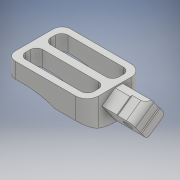
# Autodesk Inventor part: FootpegLeft
Saved by Autodesk Inventor 2018 (Build 220112000, 112)
## iProperties
Created: 2018-01-01
Part Number: FootpegLeft
Material: Generic
Document SubType Name: Modeling
Designer: eroldan
Density: 1 g/cm^3
Appearance: Default
Author: eroldan
Autodesk Inventor part; units mm, degrees
ref_plane "YZ Plane" through (0, 0, 0) normal (1, 0, 0) x (0, 1, 0)
ref_plane "XZ Plane" through (0, 0, 0) normal (0, 1, 0) x (-1, 0, 0)
ref_plane "XY Plane" through (0, 0, 0) normal (0, 0, 1) x (1, 0, 0)
sketch "Sketch1" plane through (0, 0, 0) normal (0, 0, 1) x (1, 0, 0)
  line L0 (-32.5, -28.6) -> (29.5, -28.6)
  line L1 (41.5, -16.6) -> (41.5, 16.6)
  line L2 (29.5, 28.6) -> (-32.5, 28.6)
  line L3 (-41.5, 19.6) -> (-41.5, -19.6)
  line L4 (-41.5, -28.6) -> (41.5, 28.6) construction
  line L5 (41.5, -28.6) -> (-41.5, 28.6) construction
  arc A0 (-32.5, 28.6) -> (-41.5, 19.6) centre (-32.5, 19.6) ccw
  arc A1 (-41.5, -19.6) -> (-32.5, -28.6) centre (-32.5, -19.6) ccw
  arc A2 (41.5, 16.6) -> (29.5, 28.6) centre (29.5, 16.6) ccw
  arc A3 (29.5, -28.6) -> (41.5, -16.6) centre (29.5, -16.6) ccw
  line L6 (-28.5, 21.72) -> (28.5, 21.72)
  line L7 (35, 15.22) -> (35, 10.62)
  line L8 (28.5, 4.12) -> (-28.5, 4.12)
  line L9 (-35, 10.62) -> (-35, 15.22)
  line L10 (-35, 21.72) -> (35, 4.12) construction
  line L11 (35, 21.72) -> (-35, 4.12) construction
  arc A4 (-28.5, 21.72) -> (-35, 15.22) centre (-28.5, 15.22) ccw
  arc A5 (35, 15.22) -> (28.5, 21.72) centre (28.5, 15.22) ccw
  arc A6 (28.5, 4.12) -> (35, 10.62) centre (28.5, 10.62) ccw
  arc A7 (-35, 10.62) -> (-28.5, 4.12) centre (-28.5, 10.62) ccw
  line L12 (-57.2181, 0) -> (75.1469, 0) construction
  line L13 (-28.5, -21.72) -> (28.5, -21.72)
  line L14 (35, -15.22) -> (35, -10.62)
  line L15 (28.5, -4.12) -> (-28.5, -4.12)
  line L16 (-35, -10.62) -> (-35, -15.22)
  line L17 (-35, -21.72) -> (35, -4.12) construction
  line L18 (35, -21.72) -> (-35, -4.12) construction
  arc A8 (-35, -15.22) -> (-28.5, -21.72) centre (-28.5, -15.22) ccw
  arc A9 (28.5, -21.72) -> (35, -15.22) centre (28.5, -15.22) ccw
  arc A10 (35, -10.62) -> (28.5, -4.12) centre (28.5, -10.62) ccw
  arc A11 (-28.5, -4.12) -> (-35, -10.62) centre (-28.5, -10.62) ccw
  point P0 (0, 0)
  point P1 (0, 12.92)
  point P2 (-32.5, -19.6)
  point P3 (0, -12.92)
  dimension "d0" = 83
  dimension "d1" = 57.2
  dimension "d2" = 9
  dimension "d3" = 12
  dimension "d4" = 70
  dimension "d5" = 17.6
  dimension "d6" = 6.88
  dimension "d7" = 6.5
  constraints: 38 end point, 24 point on circle, 24 point on line, 19 symmetric about line, 16 tangent, 12 centre point, 6 midpoint, 5 equal radius, 4 parallel, 3 horizontal, 2 perpendicular, 4 other
  measures "d0" distance of L5.end L4.end
  measures "d1" distance of L4.end L5.start
  measures "d2" radius of A0
  measures "d3" radius of A2
  measures "d4" distance of L10.end L11.end
  measures "d5" distance of L11.start L10.end
  measures "d6" distance between parallel lines of L6 L2
  measures "d7" radius of A4
extrude "Extrusion1" add sketch "Sketch1" against normal blind 31.75
sketch "Sketch2" plane through (41.5, -16.6, 0) normal (1, 0, 0) x (0, 0, -1)
  line L0 (0, 45.2) -> (0, 33.2) construction
  line L1 (0, 45.2) -> (31.75, 45.2) construction
  line L2 (0, 0) -> (0, -12) construction
  line L3 (0, -12) -> (31.75, -12) construction
  line L4 (0, -12) -> (22, -12)
  line L5 (0, 45.2) -> (22, 45.2)
  line L6 (31.75, 33.2) -> (31.75, 0) construction
  arc A0 (22, -12) -> (22, 45.2) centre (-15.0717, 16.6) ccw
  line L7 (0, -12) -> (0, 45.2)
  point P0 (0, 16.6)
  dimension "d10" = 22
  dimension "d11" = 22
  constraints: 6 end point, 2 point on circle, 2 point on line, 1 centre point, 1 collinear, 1 tangent
  measures "d10" distance of L2.end L4.end
  measures "d11" distance of L0.start L5.end
extrude "Extrusion2" cut sketch "Sketch2" against normal through all keep common part
sketch "Sketch3" plane through (41.5, -16.6, 0) normal (1, 0, 0) x (0, 0, -1)
  line L0 (0, -38.0508) -> (0, 74.2562) construction
  line L1 (-6.9276, -9.2387) -> (28.6783, 15.6928) construction
  line L2 (10.7388, 3.1315) -> (-2.4534, 21.972)
  line L3 (-2.4534, 21.972) -> (15.486, 34.5333)
  line L4 (20.3605, 33.6738) -> (29.5378, 20.5674)
  arc A0 (28.6783, 15.6928) -> (29.5378, 20.5674) centre (26.6707, 18.5598) ccw
  arc A1 (20.3605, 33.6738) -> (15.486, 34.5333) centre (17.4935, 31.6663) ccw
  line L5 (10.7388, 3.1315) -> (28.6783, 15.6928)
  point P0 (0, 16.6)
  point P1 (31.5453, 17.7003)
  point P2 (18.353, 36.5408)
  dimension "d15" = 25.4
  dimension "d16" = 23
  dimension "d24" = 3.5
  dimension "d42" = 55
  constraints: 12 end point, 5 point on line, 5 tangent, 4 point on circle, 2 centre point, 1 equal radius, 1 parallel, 1 vertical
  measures "d15" distance of point (31.545, 17.7) L2.start
  measures "d16" distance of L2.start L2.end
  measures "d24" radius of A0
  measures "d42" angle of L1 L0
extrude "Extrusion3" add sketch "Sketch3" along normal blind 31.75
sketch "Sketch4" plane through (73.25, -16.6, 0) normal (1, 0, 0) x (0, 0, -1)
  line L0 (0, 18.4681) -> (0, 23.6899) construction
  line L1 (-2.4534, 21.972) -> (10.7388, 3.1315) construction
  line L2 (15.486, 34.5333) -> (-2.4534, 21.972) construction
  line L3 (1.2, 16.7543) -> (1.2, 24.5301)
  line L4 (1.2, 16.7543) -> (-2.4534, 21.972)
  line L5 (1.2, 24.5301) -> (-2.4534, 21.972)
  point P0 (0, 16.6)
  point P1 (18.353, 36.5408)
  dimension "d21" = 1.2
  constraints: 6 end point, 2 point on line, 1 collinear, 1 perpendicular, 1 vertical
  measures "d21" distance between parallel lines of L3 L0
extrude "Extrusion5" cut sketch "Sketch4" against normal blind 31.75
sketch "Sketch5" plane through (41.5, -0.9072, -28.6783) normal (0, -0.819152, -0.5735764) x (1, 0, 0)
  line L0 (31.75, 6) -> (31.75, 14.7)
  line L1 (31.75, -3.5) -> (31.75, 0) construction
  line L2 (31.75, 21.9) -> (31.75, 0) construction
  line L3 (0, 21.9) -> (31.75, 21.9) construction
  line L4 (24.55, 21.9) -> (15.63, 21.9)
  line L5 (0, 32.4929) -> (0, 8.9762) projected
  arc A0 (31.75, 14.7) -> (24.55, 21.9) centre (24.55, 14.7) ccw construction
  line L6 (15.63, 20.7) -> (24.55, 20.7)
  arc A1 (30.55, 14.7) -> (24.55, 20.7) centre (24.55, 14.7) ccw
  line L7 (30.55, 14.7) -> (30.55, 6)
  line L8 (30.55, 6) -> (31.75, 6)
  line L9 (15.63, 20.7) -> (15.63, 21.9)
  line L10 (24.55, 21.9) -> (31.75, 21.9)
  line L11 (31.75, 21.9) -> (31.75, 14.7)
  point P0 (-41.5, 22.9715)
  dimension "d25" = 9.5
  dimension "d26" = 15.63
  dimension "d27" = 7.2
  dimension "d28" = 1.2
  constraints: 16 end point, 4 point on circle, 4 tangent, 3 point on line, 2 centre point, 2 collinear, 1 horizontal, 1 perpendicular, 1 vertical, 2 other
  measures "d25" distance of L1.start L0.start
  measures "d26" distance from line of L5 L4.end
  measures "d27" radius of A0
  measures "d28" radial gap between concentric circles of A0 A1
extrude "Extrusion6" cut sketch "Sketch5" against normal blind 31.75
sketch "Sketch6" plane through (41.5, -16.6, 0) normal (-1, 0, 0) x (0, 0, 1)
  line L0 (-1.2, 18.8465) -> (-1.2, 24.5301) projected
  line L1 (-1.2, 24.5301) -> (-3.4445, 26.1017) projected
  line L2 (-3.4445, 26.1017) -> (-10.5711, 31.0918) projected
  line L3 (-15.486, 34.5333) -> (-10.5711, 31.0918) projected
  arc A0 (-15.486, 34.5333) -> (-20.3605, 33.6738) centre (-17.4935, 31.6663) ccw projected
  line L4 (-29.5378, 20.5674) -> (-20.3605, 33.6738) projected
  arc A1 (-29.5378, 20.5674) -> (-28.6783, 15.6928) centre (-26.6707, 18.5598) ccw projected
  line L5 (-23.7633, 12.2513) -> (-28.6783, 15.6928) projected
  line L6 (-16.6367, 7.2612) -> (-11.7218, 3.8198) projected
  line L7 (-23.7633, 12.2513) -> (-16.6367, 7.2612) projected
  line L8 (-11.7218, 3.8198) -> (-10.7388, 3.1315) projected
  line L9 (-10.7388, 3.1315) -> (-1.2, 16.7543) projected
  line L10 (-1.2, 16.7543) -> (-1.2, 18.8465) projected
  point P0 (0, 16.6)
extrude "Extrusion7" add sketch "Sketch6" along normal up to surface (6.5 mm away)
sketch "Sketch7" plane through (41.5, -0.9072, -28.6783) normal (0, -0.819152, -0.5735764) x (1, 0, 0)
  line L0 (30.55, 6) -> (30.55, 14.7) projected
  line L1 (24.55, 20.7) -> (15.63, 20.7) projected
  point P0 (-41.5, 22.9715)
  point P1 (19.35, 8.7)
  dimension "d33" = 11.2
  dimension "d34" = 12
  measures "d33" distance from line of L0 point (19.35, 8.7)
  measures "d34" distance from line of L1 point (19.35, 8.7)
hole "Hole1" at (60.85, -5.8973, -21.5516) direction (0, 0.819152, 0.5735764) diameter 8.5 end through all
sketch "Sketch8" plane through (-32.5, 28.6, 0) normal (0, 1, 0) x (1, 0, 0)
  line L0 (-9, 0) -> (-9, 27.4502) projected
  line L1 (-9, 27.4502) -> (-9, 31.75) projected
  line L2 (0, 22) -> (62, 22) construction
  line L3 (-9, 16) -> (13, 16)
  line L4 (74, 31.75) -> (60.9017, 31.75)
  arc A0 (13, 16) -> (59.2594, 31.2605) centre (7.523, 110.346) ccw
  arc A1 (60.9017, 31.75) -> (59.2594, 31.2605) centre (60.9017, 28.75) ccw
  line L5 (74, 0) -> (-9, 0)
  line L6 (74, 0) -> (110.0916, 0)
  line L7 (110.0916, 0) -> (110.0916, 31.75)
  line L8 (110.0916, 31.75) -> (74, 31.75)
  point P0 (32.5, 0)
  point P1 (60, 31.75)
  dimension "d44" = 16
  dimension "d45" = 22
  dimension "d46" = 14
  dimension "d47" = 3
  constraints: 12 end point, 5 point on circle, 4 horizontal, 2 centre point, 2 point on line, 2 tangent, 1 collinear, 1 perpendicular
  measures "d44" distance of L3.start L0.start
  measures "d45" distance of L3.start L3.end
  measures "d46" distance of L4.start point (60, 31.75)
  measures "d47" radius of A1
extrude "Extrusion8" cut sketch "Sketch8" against normal through all keep common part
body "Solid1"
